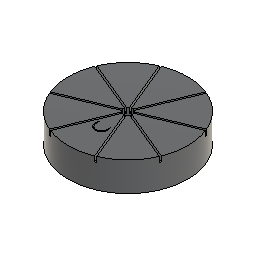
RGB_ChristmasLight_Base_Enclosure_Top_v1 (Autodesk Fusion 360 design; units mm, degrees)
Autodesk Fusion 360 part; units mm, degrees
note: some values were not read from the file. Set by a fixed rule: which sketch regions a step uses.
sketch "Sketch1" plane through (0, 0, 0) normal (0, 0, 1) x (1, 0, 0)
  circle A0 centre (0, 0) radius 30 construction
  circle A1 centre (0, 0) radius 32
  circle A2 centre (0, 0) radius 34
  dimension "d10" = 60
  dimension "d11" = 2
  dimension "d12" = 4
  constraint coincident A0.centre A1.centre
  measures "d10" diameter of A0
extrude "Extrude1" add sketch "Sketch1" along normal blind 16.6 contours A1 | A2
extrude "Extrude2" cut sketch "Sketch1" along normal blind 12.6 contours A1
sketch "Sketch2" plane through (0, 0, 16.6) normal (0, 0, 1) x (-1, 0, 0)
  circle A0 centre (0, 0) radius 34
  circle A1 centre (0, 0) radius 2.75
  line L0 (0, 0) -> (0, 15) construction
  circle A2 centre (0, 15) radius 3.65
  line L1 (0, 0) -> (-13.0112, 31.4119) construction
  line L2 (0, 0) -> (34, 0) construction
  line L3 (0.4619, 0.1913) -> (-12.5493, 31.6032)
  line L4 (-0.4619, -0.1913) -> (-13.4732, 31.2206)
  line L5 (0.5729, 2.6897) -> (12.5493, 31.6032)
  line L6 (1.4968, 2.307) -> (13.4732, 31.2206)
  line L7 (2.307, 1.4968) -> (31.2206, 13.4732)
  line L8 (2.6897, 0.5729) -> (31.6032, 12.5493)
  line L9 (2.6897, -0.5729) -> (31.6032, -12.5493)
  line L10 (2.307, -1.4968) -> (31.2206, -13.4732)
  line L11 (1.4968, -2.307) -> (13.4732, -31.2206)
  line L12 (0.5729, -2.6897) -> (12.5493, -31.6032)
  line L13 (-0.5729, -2.6897) -> (-12.5493, -31.6032)
  line L14 (-1.4968, -2.307) -> (-13.4732, -31.2206)
  line L15 (-2.307, -1.4968) -> (-31.2206, -13.4732)
  line L16 (-2.6897, -0.5729) -> (-31.6032, -12.5493)
  line L17 (-2.6897, 0.5729) -> (-31.6032, 12.5493)
  line L18 (-2.307, 1.4968) -> (-31.2206, 13.4732)
  circle A3 centre (0, 15) radius 3.15
  line L19 (3.1499, 14.9727) -> (3.1339, 13.1289)
  line L20 (-3.15, 15) -> (-3.15, 13.1561)
  dimension "d35" = 5.5
  dimension "d38" = 15
  dimension "d39" = 7.3
  dimension "d42" = 112.5
  dimension "d43" = 34
  dimension "d50" = 0.5
  dimension "d51" = -0.5
  dimension "d96" = -0.5
  constraint coincident A0.centre A1.centre
  constraint vertical L0
  constraint coincident L0.end A2.centre
  constraint horizontal L2
  constraint coincident A1 L5.start
  constraint coincident A1 L6.start
  constraint coincident A1 L7.start
  constraint coincident A1 L8.start
  constraint coincident A1 L9.start
  constraint coincident A1 L10.start
  constraint coincident A1 L11.start
  constraint coincident A1 L12.start
  constraint coincident A1 L13.start
  constraint coincident A1 L14.start
  constraint coincident A1 L15.start
  constraint coincident A1 L16.start
  constraint coincident A1 L17.start
  constraint coincident A1 L18.start
  constraint coincident A3 L19.start
  constraint coincident A2 L19.end
  constraint tangent A3 L19
  constraint coincident A3 L20.start
  constraint coincident A2 L20.end
  constraint tangent A3 L20
  constraint parallel L0 L20
  measures "d35" diameter of A1
  measures "d38" distance of A0.centre L0.end
  measures "d39" diameter of A2
  measures "d42" angle of L1 L2
  measures "d43" distance of A0.centre L1.end
extrude "Extrude3" cut sketch "Sketch2" against normal blind 4 contours A1
extrude "Extrude4" cut sketch "Sketch2" against normal blind 4 contours A2 A3 L19 L20 | A2 A3 L19 L20 | A3
extrude "Extrude6" cut sketch "Sketch2" against normal blind 3 contours A0 A1 L7 L8 | A0 A1 L9 L10 | A0 A1 L5 L6 | A0 A1 L11 L12 | A0 A1 L3 L4 | A0 A1 L13 L14 | A0 A1 L17 L18 | A0 A1 L15 L16
extrude "Extrude7" add sketch "Sketch2" against normal blind 0.5 contours A2 A3 L19 L20 | A3 picked at (0.2428, 11.5318)
sketch "Sketch3" plane through (0, 0, 12.6) normal (0, 0, -1) x (1, 0, 0)
  circle A0 centre (0, 15) radius 3.65
  circle A1 centre (0, 0) radius 2.75
  circle A2 centre (0, 0) radius 32
  circle A3 centre (0, 0) radius 25 construction
  line L0 (0, 0) -> (0, 25) construction
  line L1 (0, 25) -> (0, 22) construction
  circle A4 centre (0, 25) radius 1.6
  arc A5 (0, 22) -> (2.1213, 22.8787) centre (0, 25) ccw
  line L2 (2.1213, 22.8787) -> (9.7281, 30.4855)
  line L3 (2.1213, 22.8787) -> (12.8789, 22.8787) construction
  line L4 (-2.1213, 22.8787) -> (-9.7281, 30.4855)
  arc A6 (-2.1213, 22.8787) -> (0, 22) centre (0, 25) ccw
  circle A7 centre (-21.6506, -12.5) radius 1.6
  line L5 (-20.8742, -9.6022) -> (-31.2652, -6.8179)
  arc A8 (-19.0526, -11) -> (-20.8742, -9.6022) centre (-21.6506, -12.5) ccw
  arc A9 (-18.7529, -13.2765) -> (-19.0526, -11) centre (-21.6506, -12.5) ccw
  line L6 (-18.7529, -13.2765) -> (-21.5371, -23.6675)
  circle A10 centre (21.6506, -12.5) radius 1.6
  line L7 (18.7529, -13.2765) -> (21.5371, -23.6675)
  arc A11 (19.0526, -11) -> (18.7529, -13.2765) centre (21.6506, -12.5) ccw
  arc A12 (20.8742, -9.6022) -> (19.0526, -11) centre (21.6506, -12.5) ccw
  line L8 (20.8742, -9.6022) -> (31.2652, -6.8179)
  dimension "d99" = -7
  dimension "d100" = 3
  dimension "d101" = 3.2
  dimension "d102" = 45
  dimension "d104" = 360
  constraint coincident A1.centre A2.centre
  constraint coincident A3 L0.end
  constraint vertical L0
  constraint parallel L0 L1
  constraint coincident L0.end L1.start
  constraint horizontal L3
  constraint coincident A2 L2.end
  constraint tangent A5 L2
  constraint symmetric A5.start L1 A6.end
  constraint symmetric L1 A5.end L4.start
  constraint symmetric L1 A5 A6
  constraint symmetric L1 L2.end L4.end
  measures "d100" distance of L0.end L1.end
  measures "d101" diameter of A4
  measures "d102" angle of L2 L3
extrude "Extrude8" add sketch "Sketch3" along normal blind 3.45 contours A2 A5 L2 L4 A6 | A2 L7 A11 A12 L8 | A2 L5 A8 A9 L6
